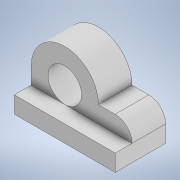
# Autodesk Inventor part: 零件4
Saved by Autodesk Inventor 2020 (Build 240168000, 168)
## iProperties
Created: 2020-09-19
Part Number: 零件4
Material: 一般
Document SubType Name: Modeling
Designer: User
Density: 1 g/cm^3
Appearance: 預設
Author: User
Autodesk Inventor part; units mm, degrees
ref_plane "YZ Plane" through (0, 0, 0) normal (1, 0, 0) x (0, 1, 0)
ref_plane "XZ Plane" through (0, 0, 0) normal (0, 1, 0) x (-1, 0, 0)
ref_plane "XY Plane" through (0, 0, 0) normal (0, 0, 1) x (1, 0, 0)
sketch "草圖1" plane through (0, 0, 0) normal (0, 0, 1) x (1, 0, 0)
  circle A0 centre (0, 0) radius 10
  arc A1 (20, 0) -> (-20, 0) centre (0, 0) ccw
  line L0 (-20, 0) -> (-20, -20)
  line L1 (-20, -20) -> (40, -20)
  line L2 (40, -20) -> (40, -10)
  line L3 (40, -10) -> (-20, -10)
  line L4 (-20, -10) -> (-20, -20)
  line L5 (20, 0) -> (30, 0)
  line L6 (40, -10) -> (40, -10)
  arc A2 (40, -10) -> (30, 0) centre (30, -10) ccw
  point P0 (40, 0)
  point P1 (0, -10)
  constraints: 14 end point, 4 point on circle, 3 centre point, 2 coincident, 2 horizontal, 2 parallel, 2 point on line, 2 tangent, 2 vertical, 1 perpendicular
extrude "擠出1" add sketch "草圖1" along normal blind 30 contours L3 L2 L1 L0
extrude "擠出2" add sketch "草圖1" along normal blind 20 contours L3 L0 A1 L5 A2
